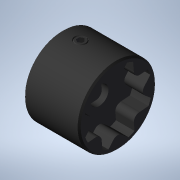
# Autodesk Inventor part: MSF-25 - 6-8 Casing 1
Saved by Autodesk Inventor 2021 (Build 250183000, 183)
## iProperties
Created: 2026-05-20
Part Number: MSF-25 - 6-8 Casing 1
Material: Generic
Catalog Web Link: www.3dfindit.com
Description: MSF left-MSF
Vendor: NBK
Document SubType Name: Modeling
Designer: psAdmin
Manufacturer: NBK
Mass: 6.66258 g
Surface Area: 31.2231 cm^2
Volume: 6.66258 cm^3
Density: 1 g/cm^3
Appearance: PSOLRGB-176-176-176
Category: PARTsolutions
Company: NBK
Title: MSF-25
Author: Cadenas PARTsolutions
Comments: MSF
PSOL_IDENT_0: {$CADENAS_DATA/23d-libs/nbk/motion_control_parts/couplicon_mini/msf/msf_left.prj},173 {VTYP=3D},{NB=
PSOL_IDENT_1: MSF-25 - 6-8 Casing 1},{LINA=MSF-25},{NN=MSF left},{DATE=08.05.2026 02:12:20},{GEOMDATE=08.12.2014 0
PSOL_IDENT_2: 8:15:56},{VERSION=},{LINEID=40},{WBVAR=D1D2},{WBNUMERIC=}  {NB=MSF-25 - 6-8 Casing 1},{LINA=MSF-25},
PSOL_IDENT_3: {KT=DUMMY},{CN=MSF-25},{D1D2=6-8},{D1D2X1='6-6','6-6.35','6-8','6-10','6-12','6.35-6.35','6.35-8','6
PSOL_IDENT_4: .35-10','6.35-12','8-8','8-10','8-12','10-10','10-12','12-12'},{A=25},{B=18},{L=12},{W=41},{F=6},{M=
PSOL_IDENT_5: M4},{WT=1.7},{C=17},{K=22},{D=10/10},{NDM=4.000},{KDM=3.242222},{P=0.700},{D1=6},{D2=8},{K1=3.760},{
PSOL_IDENT_6: DU=16.250},{BL=6.000},{H=2.000},{T=1.500}
NB: MSF-25 - 6-8 Casing 1
NN: MSF left
NT: MSF
NBSYN: $CN. - $D1D2. Casing 1
LINA: MSF-25
CATALOG: NBK (Nabeya Bi-tech Kaisha
CN: MSF-25
D1D2: 6-8
D1D2X1: '6-6','6-6.35','6-8','6-10','6-12','6.35-6.35','6.35-8','6.35-10','6.35-12','8-8','8-10','8-12','10-10','10-12','12-12'
A: 25
B: 18
L: 12
W: 41
F: 6
M: M4
WT: 1.7
C: 17
K: 22
D: 10/10
NDM: 4
P: 0.7
K1: 3.76
DU: 16.25
BL: 6
H: 2
T: 1.5
SUPPLIER: NBK
ARTICLENO: MSF-25 - 6-8 Casing 1
BOMINFO: MSF-25
CREATOR: CADENAS GmbH
Autodesk Inventor part; units mm, degrees
sketch "Sketch_1" plane through (0, 0, 0) normal (0, 0, 1) x (1, 0, 0)
  line L0 (18, 0) -> (0, 0)
  line L1 (0, 0) -> (0, 12)
  line L2 (0, 12) -> (0.5, 12.5)
  line L3 (0.5, 12.5) -> (17.5, 12.5)
  line L4 (17.5, 12.5) -> (18, 12)
  line L5 (18, 12) -> (18, 0)
  line L6 (18, 0) -> (0, 0)
  constraints: 14 end point
revolve "Revolution1" add sketch "Sketch_1" angle 360 about axis through (18, 0, 0) along (1, 0, 0)
sketch "Sketch_2" plane through (12, 0, 0) normal (1, 0, 0) x (0, 0, -1)
  line L0 (-10.681, 3.0208) -> (-8.764, 1.4122)
  arc A0 (-8.764, -1.4122) -> (-8.764, 1.4122) centre (-10.005, 0) ccw
  line L1 (-8.764, -1.4122) -> (-10.5287, -3.5153)
  arc A1 (-10.5287, -3.5153) -> (-9.6887, -5.4166) centre (0, 0) ccw
  line L2 (-9.6887, -5.4166) -> (-7.1956, -5.1985)
  arc A2 (-5.1985, -7.1956) -> (-7.1956, -5.1985) centre (-7.0746, -7.0746) ccw
  line L3 (-5.1985, -7.1956) -> (-4.9592, -9.9306)
  arc A3 (-4.9592, -9.9306) -> (-3.0208, -10.681) centre (0, 0) ccw
  line L4 (-3.0208, -10.681) -> (-1.4122, -8.764)
  arc A4 (1.4122, -8.764) -> (-1.4122, -8.764) centre (0, -10.005) ccw
  line L5 (1.4122, -8.764) -> (3.5153, -10.5287)
  arc A5 (3.5153, -10.5287) -> (5.4166, -9.6887) centre (0, 0) ccw
  line L6 (5.4166, -9.6887) -> (5.1985, -7.1956)
  arc A6 (7.1956, -5.1985) -> (5.1985, -7.1956) centre (7.0746, -7.0746) ccw
  line L7 (7.1956, -5.1985) -> (9.9306, -4.9592)
  arc A7 (9.9306, -4.9592) -> (10.681, -3.0208) centre (0, 0) ccw
  line L8 (10.681, -3.0208) -> (8.764, -1.4122)
  arc A8 (8.764, 1.4122) -> (8.764, -1.4122) centre (10.005, 0) ccw
  line L9 (8.764, 1.4122) -> (10.5287, 3.5153)
  arc A9 (10.5287, 3.5153) -> (9.6887, 5.4166) centre (0, 0) ccw
  line L10 (9.6887, 5.4166) -> (7.1956, 5.1985)
  arc A10 (5.1985, 7.1956) -> (7.1956, 5.1985) centre (7.0746, 7.0746) ccw
  line L11 (5.1985, 7.1956) -> (4.9592, 9.9306)
  arc A11 (4.9592, 9.9306) -> (3.0208, 10.681) centre (0, 0) ccw
  line L12 (3.0208, 10.681) -> (1.4122, 8.764)
  arc A12 (-1.4122, 8.764) -> (1.4122, 8.764) centre (0, 10.005) ccw
  line L13 (-1.4122, 8.764) -> (-3.5153, 10.5287)
  arc A13 (-3.5153, 10.5287) -> (-5.4166, 9.6887) centre (0, 0) ccw
  line L14 (-5.4166, 9.6887) -> (-5.1985, 7.1956)
  arc A14 (-7.1956, 5.1985) -> (-5.1985, 7.1956) centre (-7.0746, 7.0746) ccw
  line L15 (-7.1956, 5.1985) -> (-9.9306, 4.9592)
  arc A15 (-9.9306, 4.9592) -> (-10.681, 3.0208) centre (0, 0) ccw
  constraints: 32 end point, 32 point on circle, 16 centre point
extrude "Extrusion1" cut sketch "Sketch_2" along normal blind 6
sketch "Sketch_3" plane through (0, 0, 0) normal (1, 0, 0) x (0, 1, 0)
  circle A0 centre (0, 0) radius 3
  constraints: 1 centre point
extrude "Extrusion2" cut sketch "Sketch_3" along normal mid plane 34
sketch "Sketch_4" plane through (0, 0, 0) normal (0, 0, 1) x (1, 0, 0)
  line L0 (6, 0) -> (6, 12.5)
  line L1 (6, 12.5) -> (8, 12.5)
  line L2 (8, 12.5) -> (7.6211, 12.1211)
  line L3 (7.6211, 12.1211) -> (7.6211, 0.3789)
  line L4 (7.6211, 0.3789) -> (8, 0)
  line L5 (8, 0) -> (6, 0)
  line L6 (6, 0) -> (6, 12.5)
  constraints: 14 end point
revolve "Revolution2" cut sketch "Sketch_4" angle 360 about axis through (6, 0, 0) along (0, -1, 0)
sketch "Sketch_6" plane through (0, 0, 0) normal (0, 1, 0) x (-1, 0, 0)
  line L0 (-6, 0) -> (-6, -12.5)
  line L1 (-6, -12.5) -> (-8, -12.5)
  line L2 (-8, -12.5) -> (-7.6211, -12.1211)
  line L3 (-7.6211, -12.1211) -> (-7.6211, -0.3789)
  line L4 (-7.6211, -0.3789) -> (-8, 0)
  line L5 (-8, 0) -> (-6, 0)
  line L6 (-6, 0) -> (-6, -12.5)
  constraints: 14 end point
revolve "Revolution3" cut sketch "Sketch_6" angle 360 about axis through (6, 0, 0) along (0, 0, 1)
sketch "Sketch_8" plane through (0, 0, 0) normal (0, 0, 1) x (1, 0, 0)
  line L0 (6, 6.5) -> (6, 12.5)
  line L1 (6, 12.5) -> (7.6211, 12.5)
  line L2 (7.6211, 12.5) -> (8, 12.1211)
  line L3 (8, 12.1211) -> (8, 6.8789)
  line L4 (8, 6.8789) -> (7.6211, 6.5)
  line L5 (7.6211, 6.5) -> (6, 6.5)
  line L6 (6, 6.5) -> (6, 12.5)
  constraints: 14 end point
revolve "Revolution4" add sketch "Sketch_8" angle 360 about axis through (6, 6.5, 0) along (0, -1, 0)
sketch "Sketch_5" plane through (0, 11, 0) normal (0, 1, 0) x (1, 0, 0)
  line L0 (5, -0.5774) -> (6, -1.1547)
  line L1 (6, -1.1547) -> (7, -0.5774)
  line L2 (7, -0.5774) -> (7, 0.5774)
  line L3 (7, 0.5774) -> (6, 1.1547)
  line L4 (6, 1.1547) -> (5, 0.5774)
  line L5 (5, 0.5774) -> (5, -0.5774)
  constraints: 12 end point
extrude "Extrusion3" cut sketch "Sketch_5" along normal blind 1.5
sketch "Sketch_7" plane through (0, 0, 0) normal (0, 1, 0) x (-1, 0, 0)
  line L0 (-6, -6.5) -> (-6, -12.5)
  line L1 (-6, -12.5) -> (-7.6211, -12.5)
  line L2 (-7.6211, -12.5) -> (-8, -12.1211)
  line L3 (-8, -12.1211) -> (-8, -6.8789)
  line L4 (-8, -6.8789) -> (-7.6211, -6.5)
  line L5 (-7.6211, -6.5) -> (-6, -6.5)
  line L6 (-6, -6.5) -> (-6, -12.5)
  constraints: 14 end point
revolve "Revolution5" add sketch "Sketch_7" angle 360 about axis through (6, 0, -6.5) along (0, 0, 1)
sketch "Sketch_9" plane through (0, 0, -12.5) normal (0, 0, 1) x (1, 0, 0)
  line L0 (5, -0.5774) -> (6, -1.1547)
  line L1 (6, -1.1547) -> (7, -0.5774)
  line L2 (7, -0.5774) -> (7, 0.5774)
  line L3 (7, 0.5774) -> (6, 1.1547)
  line L4 (6, 1.1547) -> (5, 0.5774)
  line L5 (5, 0.5774) -> (5, -0.5774)
  constraints: 12 end point
extrude "Extrusion4" cut sketch "Sketch_9" along normal blind 1.5
ref_plane "left_XY" through (12, 0, 0) normal (1, 0, 0) x (0, 0, -1)
ref_plane "left_YZ" through (12, 0, 0) normal (0, 0, -1) x (0, 1, 0)
ref_plane "left_ZX" through (12, 0, 0) normal (0, 1, 0) x (1, 0, 0)
ref_plane "left_dummy_XY" through (0, 0, 0) normal (1, 0, 0) x (0, 0, -1)
ref_plane "left_dummy_YZ" through (0, 0, 0) normal (0, 0, -1) x (0, 1, 0)
ref_plane "left_dummy_ZX" through (0, 0, 0) normal (0, 1, 0) x (1, 0, 0)
body "Solid1"
